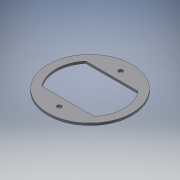
# Autodesk Inventor part: retainer
Saved by Autodesk Inventor 2018 (Build 220112000, 112)
## iProperties
Created: 2018-04-19
Part Number: retainer
Material: Generic
Document SubType Name: Modeling
Designer: Cole Tucker
Density: 1 g/cm^3
Appearance: Default
Author: Cole Tucker
Autodesk Inventor part; units mm, degrees
ref_plane "YZ Plane" through (0, 0, 0) normal (1, 0, 0) x (0, 1, 0)
ref_plane "XZ Plane" through (0, 0, 0) normal (0, 1, 0) x (-1, 0, 0)
ref_plane "XY Plane" through (0, 0, 0) normal (0, 0, 1) x (1, 0, 0)
sketch "Sketch1" plane through (0, 0, 0) normal (0, 1, 0) x (-1, 0, 0)
  circle A0 centre (0, 0) radius 24.765
  circle A1 centre (0, 0) radius 30.48
  dimension "d0" = 49.53
  dimension "d1" = 60.96
  constraints: 2 centre point, 2 coincident
  measures "d0" diameter of A0
  measures "d1" diameter of A1
extrude "Extrusion1" add sketch "Sketch1" along normal blind 1.6002
sketch "Sketch2" plane through (0, 1.6002, 0) normal (0, 1, 0) x (1, 0, 0)
  line L0 (0, 0) -> (0, 15.9004)
  line L1 (0, 15.9004) -> (-18.9864, 15.9004)
  circle A0 centre (0, 0) radius 24.765 projected
  line L2 (0, 15.9004) -> (18.9864, 15.9004)
  dimension "d4" = 15.9004
  constraints: 6 end point, 2 point on circle, 1 perpendicular, 1 point on line, 1 vertical
  measures "d4" distance of L0.start L0.end
extrude "Extrusion2" add sketch "Sketch2" against normal blind 1.6002 contours L1 A0 L2 picked at (-11.1522, 17.2995)
pattern_circular "Circular Pattern1" count 2 over 360 about axis through (0, 0, 0) along (0, 1, 0) of "Extrusion2"
sketch "Sketch3" plane through (0, 1.6002, 0) normal (0, 1, 0) x (1, 0, 0)
  circle A0 centre (0, 0) radius 30.48 projected
  line L0 (-18.9864, -15.9004) -> (18.9864, -15.9004) projected
  line L1 (0, 0) -> (0, -22.2504)
  dimension "d11" = 22.2504
  constraints: 2 end point, 1 coincident, 1 vertical
  measures "d11" distance of L1.start L1.end
hole "Hole1" at (0, 1.6002, 22.2504) direction (0, -1, 0) diameter 3.175 depth 25.4 tip angle 118
pattern_circular "Circular Pattern2" count 2 over 360 about axis through (0, 0, 0) along (0, 1, 0) of "Hole1"
body "Solid1"
